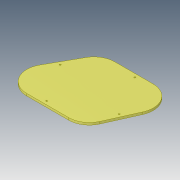
# Autodesk Inventor part: tampa traseira do corpo
Saved by Autodesk Inventor 2016 (Build 200138000, 138)
## iProperties
Created: 2018-12-06
Part Number: tampa traseira do corpo
Material: PET Plastic
Document SubType Name: Modeling
Designer: lesly
Density: 1.541 g/cm^3
Appearance: Yellow(1)
Author: lesly
Autodesk Inventor part; units mm, degrees
ref_plane "YZ Plane" through (0, 0, 0) normal (1, 0, 0) x (0, 1, 0)
ref_plane "XZ Plane" through (0, 0, 0) normal (0, 1, 0) x (-1, 0, 0)
ref_plane "XY Plane" through (0, 0, 0) normal (0, 0, 1) x (1, 0, 0)
sketch "Sketch1" plane through (0, 0, 0) normal (1, 0, 0) x (0, 1, 0)
  line L0 (0, -332) -> (-46, -332) construction
  line L1 (-46, -332) -> (-46, -297.4128)
  line L2 (-46, -332) -> (-46, -348.8838)
  line L3 (-85.3886, -374.4631) -> (-125.3109, -356.6885)
  line L4 (-141.9223, -331.1092) -> (-141.9223, -275.0602)
  arc A0 (-85.3886, -374.4631) -> (-46, -348.8838) centre (-74, -348.8838) ccw
  arc A1 (-100.2431, -250.629) -> (-141.9223, -275.0602) centre (-113.9223, -275.0602) ccw
  arc A2 (-46, -297.4128) -> (-60.3209, -272.9817) centre (-74, -297.4128) ccw
  arc A3 (-141.9223, -331.1092) -> (-125.3109, -356.6885) centre (-113.9223, -331.1092) ccw
  line L5 (0, -332) -> (-46, -332) construction
  line L6 (-46, -332) -> (-46, -297.4128)
  line L7 (-46, -332) -> (-46, -348.8838)
  line L8 (-85.3886, -374.4631) -> (-125.3109, -356.6885)
  line L9 (-141.9223, -331.1092) -> (-141.9223, -275.0602)
  arc A4 (-85.3886, -374.4631) -> (-46, -348.8838) centre (-74, -348.8838) ccw
  arc A5 (-100.2431, -250.629) -> (-141.9223, -275.0602) centre (-113.9223, -275.0602) ccw
  arc A6 (-46, -297.4128) -> (-60.3209, -272.9817) centre (-74, -297.4128) ccw
  arc A7 (-141.9223, -331.1092) -> (-125.3109, -356.6885) centre (-113.9223, -331.1092) ccw
  line L10 (0, -332) -> (-46, -332) construction
  line L11 (-46, -332) -> (-46, -297.4128)
  line L12 (-46, -332) -> (-46, -348.8838)
  line L13 (-85.3886, -374.4631) -> (-125.3109, -356.6885)
  line L14 (-141.9223, -331.1092) -> (-141.9223, -275.0602)
  line L15 (-60.3209, -272.9817) -> (-100.2431, -250.629)
  arc A8 (-85.3886, -374.4631) -> (-46, -348.8838) centre (-74, -348.8838) ccw
  arc A9 (-100.2431, -250.629) -> (-141.9223, -275.0602) centre (-113.9223, -275.0602) ccw
  arc A10 (-46, -297.4128) -> (-60.3209, -272.9817) centre (-74, -297.4128) ccw
  arc A11 (-141.9223, -331.1092) -> (-125.3109, -356.6885) centre (-113.9223, -331.1092) ccw
  line L16 (-141.8223, -275.0602) -> (-141.8223, -331.1092)
  arc A12 (-141.8223, -331.1092) -> (-125.2702, -356.5972) centre (-113.9223, -331.1092) ccw
  line L17 (-125.2702, -356.5972) -> (-85.348, -374.3717)
  arc A13 (-85.348, -374.3717) -> (-46.1, -348.8838) centre (-74, -348.8838) ccw
  line L18 (-46.1, -348.8838) -> (-46.1, -332)
  line L19 (-46.1, -332) -> (-46.1, -297.4128)
  arc A14 (-46.1, -297.4128) -> (-60.3697, -273.0689) centre (-74, -297.4128) ccw
  line L20 (-60.3697, -273.0689) -> (-100.292, -250.7163)
  arc A15 (-100.292, -250.7163) -> (-141.8223, -275.0602) centre (-113.9223, -275.0602) ccw
  point P0 (0, 0)
  point P1 (-46, -281)
  point P2 (-46, -392)
  point P3 (-141.9223, -349.2927)
  point P4 (-141.9223, -227.2927)
  point P5 (-46, -281)
  point P6 (-46, -392)
  point P7 (-141.9223, -349.2927)
  point P8 (-141.9223, -227.2927)
  point P9 (-46, -281)
  point P10 (-46, -392)
  point P11 (-141.9223, -349.2927)
  point P12 (-141.9223, -227.2927)
  dimension "d43" = 0
  dimension "d0" = 46
  dimension "d1" = 51
  dimension "d2" = 60
  dimension "d3" = 105
  dimension "d4" = 66
  dimension "d5" = 122
  dimension "d6" = 28
  dimension "d7" = 28
  dimension "d8" = 28
  dimension "d9" = 46
  dimension "d11" = 60
  dimension "d12" = 105
  dimension "d13" = 66
  dimension "d14" = 122
  dimension "d15" = 28
  dimension "d16" = 28
  dimension "d17" = 28
  dimension "d18" = 46
  dimension "d21" = 105
  dimension "d22" = 66
  dimension "d23" = 122
  dimension "d24" = 28
  dimension "d25" = 28
  dimension "d26" = 28
  dimension "d27" = 0.1
  constraints: 42 end point, 32 point on circle, 20 point on line, 20 tangent, 16 centre point, 9 vertical, 3 equal radius, 3 horizontal, 6 other
  measures "d0" distance of L0.start L1.start
  measures "d1" distance of L1.start point (-46, -281)
  measures "d2" distance of L1.start point (-46, -392)
  measures "d3" distance of point (-46, -392) point (-141.922, -349.293)
  measures "d4" angle of L2 L3
  measures "d5" distance of point (-141.922, -349.293) point (-141.922, -227.293)
  measures "d6" radius of A0
  measures "d7" radius of A1
  measures "d8" radius of A2
  measures "d9" distance of L5.start L6.start
  measures "d11" distance of L6.start point (-46, -392)
  measures "d12" distance of point (-46, -392) point (-141.922, -349.293)
  measures "d13" angle of L7 L8
  measures "d14" distance of point (-141.922, -349.293) point (-141.922, -227.293)
  measures "d15" radius of A4
  measures "d16" radius of A5
  measures "d17" radius of A6
  measures "d18" distance of L10.start L11.start
  measures "d21" distance of point (-46, -392) point (-141.922, -349.293)
  measures "d22" angle of L12 L13
  measures "d23" distance of point (-141.922, -349.293) point (-141.922, -227.293)
  measures "d24" radius of A8
  measures "d25" radius of A9
  measures "d26" radius of A10
  measures "d27" radial gap between concentric circles of A1 A15
extrude "Extrusion1" add sketch "Sketch1" along normal blind 3 contours A15 L20 A14 L19 L18 A13 L17 A12 L16
sketch "Sketch2" plane through (3, 0, 0) normal (1, 0, 0) x (0, 0, -1)
  arc A0 (250.7163, -100.292) -> (275.0602, -141.8223) centre (275.0602, -113.9223) ccw projected
  arc A1 (374.3717, -85.348) -> (348.8838, -46.1) centre (348.8838, -74) ccw projected
  arc A2 (297.4128, -46.1) -> (273.0689, -60.3697) centre (297.4128, -74) ccw projected
  arc A3 (331.1092, -141.8223) -> (356.5972, -125.2702) centre (331.1092, -113.9223) ccw projected
  circle A4 centre (328.9681, -50.7353) radius 0.5
  line L0 (273.0689, -60.3697) -> (250.7163, -100.292) projected
  circle A5 centre (264.0532, -86.152) radius 0.5
  line L1 (356.5972, -125.2702) -> (374.3717, -85.348) projected
  circle A6 centre (360.8666, -103.7379) radius 0.5
  line L2 (275.0602, -141.8223) -> (331.1092, -141.8223) projected
  circle A7 centre (296.9895, -137.1327) radius 0.5
  point P0 (0, 0)
  constraints: 4 centre point
extrude "Extrusion2" cut sketch "Sketch2" against normal blind 5
chamfer "Chamfer1" distance 0.5 angle 45 1 edges at (3, -86.152, -263.5532)
chamfer "Chamfer2" distance 0.5 angle 45 3 edges at (3, -137.1327, -296.4895) (3, -103.7379, -360.3666) (3, -50.7353, -328.4681)
body "Solid1"
